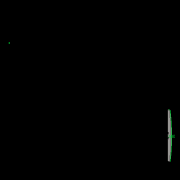
# Autodesk Inventor part: ThiccUpright
Saved by Autodesk Inventor 2021 (Build 250183000, 183)
## iProperties
Created: 2021-03-04
Part Number: ThiccUpright
Material: Steel
Document SubType Name: Modeling
Designer: Esketitttttt
Density: 7.85 g/cm^3
Appearance: Steel - Polished
Mass: 3057.13 g
Surface Area: 815.25 cm^2
Volume: 389.443 cm^3
Author: Esketitttttt
Autodesk Inventor part; units mm, degrees
ref_plane "YZ Plane" through (0, 0, 0) normal (1, 0, 0) x (0, 1, 0)
ref_plane "XZ Plane" through (0, 0, 0) normal (0, 1, 0) x (-1, 0, 0)
ref_plane "XY Plane" through (0, 0, 0) normal (0, 0, 1) x (1, 0, 0)
sketch "Sketch1" plane through (0, 0, 0) normal (0, 0, 1) x (1, 0, 0)
  line L0 (0, 0) -> (50.8, 0)
  line L1 (50.8, 0) -> (50.8, 743.1377)
  line L2 (50.8, 743.1377) -> (0, 743.1377)
  line L3 (0, 743.1377) -> (0, 0)
  arc A0 (25.4, 0) -> (25.4, 743.1377) centre (-2679.6839, 371.5689) ccw
  line L4 (0, 371.5689) -> (0, 396.9689)
  line L5 (0, 384.3401) -> (0, 308.1401)
  line L6 (0, 435.0689) -> (0, 371.5689)
  line L7 (0, 346.1689) -> (0, 371.5689)
  line L8 (0, 435.0689) -> (12.7, 435.0689)
  line L9 (12.7, 435.0689) -> (12.7, 308.0689)
  line L10 (12.7, 308.0689) -> (0, 308.0689)
  line L11 (0, 308.0689) -> (0, 435.0689)
  line L12 (0, 371.5689) -> (12.7, 371.5689)
  line L13 (12.7, 371.5689) -> (12.7, 422.3689)
  line L14 (12.7, 422.3689) -> (0, 422.3689)
  line L15 (0, 422.3689) -> (0, 371.5689)
  line L16 (0, 371.5689) -> (12.7, 371.5689)
  line L17 (12.7, 371.5689) -> (12.7, 320.7689)
  line L18 (12.7, 320.7689) -> (0, 320.7689)
  line L19 (0, 320.7689) -> (0, 371.5689)
  line L20 (0, 371.5689) -> (12.7, 371.5689)
  line L21 (12.7, 371.5689) -> (12.7, 352.5189)
  line L22 (12.7, 352.5189) -> (0, 352.5189)
  line L23 (0, 352.5189) -> (0, 371.5689)
  line L24 (0, 371.5689) -> (12.7, 371.5689)
  line L25 (12.7, 371.5689) -> (12.7, 390.6189)
  line L26 (12.7, 390.6189) -> (0, 390.6189)
  line L27 (0, 390.6189) -> (0, 371.5689)
  point P0 (0, 308.0689)
  point P1 (0, 435.0689)
  point P2 (12.7, 422.3689)
  point P3 (0, 422.3689)
  point P4 (0, 320.7689)
  point P5 (12.7, 320.7689)
  point P6 (0, 371.5689)
  point P7 (0, 320.7689)
  point P8 (0, 347.1346)
  point P9 (0, 371.5689)
  point P10 (12.7, 371.5689)
  point P11 (0, 352.5189)
  point P12 (12.7, 352.5189)
  point P13 (12.7, 390.6189)
  point P14 (0, 390.6189)
  dimension "d0" = 50.8
  dimension "d1" = 743.1377
  dimension "d13" = 12.7
  dimension "d16" = 12.7
  dimension "d17" = 12.7
  dimension "d18" = 50.8
  dimension "d19" = 50.8
  dimension "d20" = 0
  dimension "d21" = 0
  dimension "d22" = 12.7
  dimension "d23" = 12.7
  dimension "d24" = 371.5689
  dimension "d25" = 12.7
  dimension "d26" = 19.05
  dimension "d27" = 12.7
  dimension "d28" = 19.05
  constraints: 56 end point, 12 parallel, 6 horizontal, 6 perpendicular, 2 midpoint, 2 point on circle, 1 centre point, 1 point on line, 1 tangent
  measures "d0" distance of L2.end L1.end
  measures "d1" distance of L1.end L0.end
  measures "d13" distance of L9.end L10.end
  measures "d16" distance of L14.end L13.end
  measures "d17" distance of L17.end L18.end
  measures "d18" distance of L16.end L17.end
  measures "d19" distance between parallel lines of L12 L14
  measures "d20" distance between parallel lines of L5 L19
  measures "d21" distance between parallel lines of L3 L11
  measures "d22" distance between parallel lines of L10 L18
  measures "d23" distance between parallel lines of L14 L8
  measures "d24" distance of L0.start L4.start
  measures "d25" distance of L21.end L22.end
  measures "d26" distance of L20.end L21.end
  measures "d27" distance of L26.end L25.end
  measures "d28" distance of L25.end L24.end
extrude "Extrusion1" add sketch "Sketch1" along normal blind 12.7 contours L3 L10 L9 L8 L2 A0 L0 | L3 L18 L9 L10 | L22 L3 L12 L9 | L8 L9 L14 L3 | L12 L3 L26 L9
sketch "Sketch2" plane through (0, 0, 0) normal (0, 0, -1) x (-1, 0, 0)
  line L0 (0, 320.7689) -> (0, 0) projected
  line L1 (-12.7, 320.7689) -> (0, 320.7689) projected
  line L2 (-12.7, 352.5189) -> (-12.7, 320.7689) projected
  line L3 (0, 352.5189) -> (-12.7, 352.5189) projected
  line L4 (0, 390.6189) -> (0, 352.5189) projected
  line L5 (-12.7, 390.6189) -> (0, 390.6189) projected
  line L6 (-12.7, 422.3689) -> (-12.7, 390.6189) projected
  line L7 (0, 422.3689) -> (-12.7, 422.3689) projected
  line L8 (0, 743.1377) -> (0, 422.3689) projected
  line L9 (-25.4, 743.1377) -> (0, 743.1377) projected
  arc A0 (-25.4, 743.1377) -> (-25.4, 0) centre (2679.6839, 371.5689) ccw projected
  line L10 (0, 0) -> (-25.4, 0) projected
  arc A1 (-14.3025, 730.4377) -> (-14.3025, 12.7) centre (2679.6839, 371.5689) ccw
  line L11 (-14.3025, 730.4377) -> (-12.7, 730.4377)
  line L12 (-12.7, 730.4377) -> (-12.7, 435.0689)
  line L13 (-12.7, 435.0689) -> (-25.4, 435.0689)
  line L14 (-25.4, 435.0689) -> (-25.4, 377.9189)
  line L15 (-25.4, 377.9189) -> (-12.7, 377.9189)
  line L16 (-12.7, 377.9189) -> (-12.7, 365.2189)
  line L17 (-12.7, 365.2189) -> (-25.4, 365.2189)
  line L18 (-25.4, 365.2189) -> (-25.4, 308.0689)
  line L19 (-25.4, 308.0689) -> (-12.7, 308.0689)
  line L20 (-12.7, 308.0689) -> (-12.7, 12.7)
  line L21 (-12.7, 12.7) -> (-14.3025, 12.7)
  dimension "d29" = 12.7
  constraints: 22 end point, 2 point on circle, 1 centre point, 11 other
  measures "d29" radial gap between concentric circles of A0 A1
equation "\"d24\" = 0.5 * d1"
body "Solid1"
